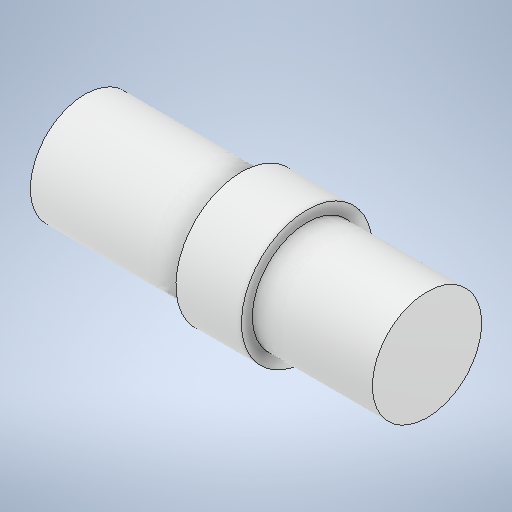
# Autodesk Inventor part: Welle_für_Kettenzug
Saved by Autodesk Inventor 2025.2 (Build 292293000, 293)
## iProperties
Created: 2025-02-03
Part Number: Welle_für_Kettenzug
Material: Generisch
Document SubType Name: Modeling
Designer: unter
Density: 1 g/cm^3
Appearance: Vorgabe
Author: unter
Autodesk Inventor part; units mm, degrees
ref_plane "YZ Plane" through (0, 0, 0) normal (1, 0, 0) x (0, 1, 0)
ref_plane "XZ Plane" through (0, 0, 0) normal (0, 1, 0) x (-1, 0, 0)
ref_plane "XY Plane" through (0, 0, 0) normal (0, 0, 1) x (1, 0, 0)
derived "Skelett_Laufkatze.ipt"
sketch "Kettenzug_welle" plane through (-97, 65, 62.4) normal (0, 0, -1) x (-1, 0, 0)
  line L0 (34, -46.5) -> (84, -46.5) construction
  line L1 (34, -83.5) -> (84, -83.5) construction
  line L2 (17, -65) -> (111, -65)
  line L3 (17, -65) -> (17, -50)
  line L4 (17, -50) -> (50, -50)
  line L5 (50, -50) -> (50, -47)
  line L6 (50, -47) -> (68, -47)
  line L7 (68, -47) -> (68, -50)
  line L8 (68, -50) -> (111, -50)
  line L9 (111, -50) -> (111, -65)
  point P0 (-97, -65)
revolve "Welle_Kettenzug" add sketch "Kettenzug_welle" angle 360 about axis through (-114, 0, 62.4) along (-1, 0, 0)
